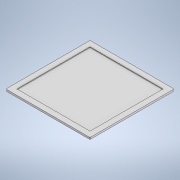
# Autodesk Inventor part: MouldBase20
Saved by Autodesk Inventor 2020.3 (Build 243373010, 373A)
## iProperties
Created: 2020-10-26
Part Number: MouldBase20
Material: Generic
Document SubType Name: Modeling
Designer: Naude Conradie
Density: 1 g/cm^3
Appearance: Default
Author: Naude Conradie
Autodesk Inventor part; units mm, degrees
ref_plane "YZ Plane" through (0, 0, 0) normal (1, 0, 0) x (0, 1, 0)
ref_plane "XZ Plane" through (0, 0, 0) normal (0, 1, 0) x (-1, 0, 0)
ref_plane "XY Plane" through (0, 0, 0) normal (0, 0, 1) x (1, 0, 0)
sketch "Sketch1" plane through (0, 0, 0) normal (0, 1, 0) x (-1, 0, 0)
  line L0 (0, 0) -> (230, 0)
  line L1 (230, 0) -> (230, -230)
  line L2 (230, -230) -> (0, -230)
  line L3 (0, -230) -> (0, 0)
  dimension "d0" = 230
  dimension "d1" = 230
  constraints: 8 end point, 2 parallel, 1 horizontal, 1 perpendicular
  measures "d0" distance of L1.end L2.end
  measures "d1" distance of L0.end L1.end
extrude "Extrusion1" add sketch "Sketch1" along normal blind 5
sketch "Sketch2" plane through (0, 5, 0) normal (0, 1, 0) x (1, 0, 0)
  line L0 (-215, 215) -> (-15, 215)
  line L1 (-15, 215) -> (-15, 15)
  line L2 (-15, 15) -> (-215, 15)
  line L3 (-215, 15) -> (-215, 215)
  line L4 (-230, 230) -> (-230, 0) projected
  point P0 (0, 0)
  dimension "d4" = 200
  dimension "d5" = 200
  dimension "d6" = 15
  dimension "d7" = 15
  constraints: 8 end point, 2 parallel, 1 horizontal, 1 perpendicular
  measures "d4" distance of L1.end L2.end
  measures "d5" distance of L0.end L1.end
  measures "d6" distance from line of L4 L0.start
  measures "d7" distance from line of L0 L4.start
extrude "Extrusion2" cut sketch "Sketch2" against normal blind 2
chamfer "Chamfer1" distance 2 angle 45 4 edges at (-230, 2.5, 0) (-230, 2.5, -230) (0, 2.5, -230) (0, 2.5, 0)
body "Solid1"
